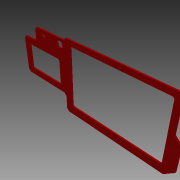
# Autodesk Inventor part: front_panel_frame
Saved by Autodesk Inventor 2014 (Build 180170000, 170)
## iProperties
Created: 2014-03-23
Part Number: front_panel_frame
Material: ABS Plastic
Document SubType Name: Modeling
Designer: buben
Density: 1.06 g/cm^3
Appearance: Smooth - Red
Author: buben
Autodesk Inventor part; units mm, degrees
ref_plane "YZ Plane" through (0, 0, 0) normal (1, 0, 0) x (0, 1, 0)
ref_plane "XZ Plane" through (0, 0, 0) normal (0, 1, 0) x (-1, 0, 0)
ref_plane "XY Plane" through (0, 0, 0) normal (0, 0, 1) x (1, 0, 0)
sketch "Sketch1" plane through (0, 0, 0) normal (0, 1, 0) x (-1, 0, 0)
  line L0 (0, -41) -> (-67, -41)
  line L1 (-67, -41) -> (-67, 0)
  line L2 (-67, 0) -> (0, 0)
  line L3 (0, 0) -> (0, -41)
  line L4 (-90, -68) -> (-242, -68)
  line L5 (-242, -68) -> (-242, 28)
  line L6 (-242, 28) -> (-90, 28)
  line L7 (-90, 28) -> (-90, -68)
  line L8 (11, -47.5) -> (11, 6.5)
  line L9 (7, 10.5) -> (-74, 10.5)
  line L10 (-78, 14.5) -> (-78, 32.5)
  line L11 (-82, 36.5) -> (-246, 36.5)
  line L12 (-250, 32.5) -> (-250, -77.5)
  line L13 (-246, -81.5) -> (-82, -81.5)
  line L14 (-78, -77.5) -> (-78, -55.5)
  line L15 (-74, -51.5) -> (7, -51.5)
  line L16 (11, -47.5) -> (7, -51.5)
  line L17 (-74, -51.5) -> (-78, -55.5)
  line L18 (-78, -77.5) -> (-82, -81.5)
  line L19 (-246, -81.5) -> (-250, -77.5)
  line L20 (-250, 32.5) -> (-246, 36.5)
  line L21 (-82, 36.5) -> (-78, 32.5)
  line L22 (-78, 14.5) -> (-74, 10.5)
  line L23 (7, 10.5) -> (11, 6.5)
  line L24 (6, -46.5) -> (-73, -46.5) construction
  line L25 (-73, -46.5) -> (-73, 5.5) construction
  line L26 (-73, 5.5) -> (6, 5.5) construction
  line L27 (6, 5.5) -> (6, -46.5) construction
  line L28 (-83, -76.5) -> (-245, -76.5) construction
  line L29 (-245, -76.5) -> (-245, 31.5) construction
  line L30 (-245, 31.5) -> (-83, 31.5) construction
  line L31 (-83, 31.5) -> (-83, -76.5) construction
  point P0 (11, 10.5)
  point P1 (-78, 10.5)
  point P2 (-78, 36.5)
  point P3 (-250, 36.5)
  point P4 (-250, -81.5)
  point P5 (-78, -81.5)
  point P6 (-78, -51.5)
  point P7 (11, -51.5)
  point P8 (-33.5, -46.5)
  point P9 (-33.5, -41)
  point P10 (6, -20.5)
  point P11 (0, -20.5)
  point P12 (-83, -22.5)
  point P13 (-90, -20)
  point P14 (-164, -76.5)
  point P15 (-166, -68)
  dimension "d0" = 67
  dimension "d1" = 41
  dimension "d2" = 152
  dimension "d3" = 96
  dimension "d4" = 4
  dimension "d5" = 4
  dimension "d6" = 4
  dimension "d7" = 4
  dimension "d8" = 4
  dimension "d9" = 4
  dimension "d10" = 4
  dimension "d11" = 4
  dimension "d12" = 4
  dimension "d13" = 4
  dimension "d14" = 4
  dimension "d15" = 4
  dimension "d16" = 4
  dimension "d17" = 4
  dimension "d18" = 4
  dimension "d19" = 4
  dimension "d20" = 79
  dimension "d21" = 52
  dimension "d22" = 162
  dimension "d23" = 108
  dimension "d24" = 10
  dimension "d25" = 26
  dimension "d26" = 5
  dimension "d27" = 5
  dimension "d28" = 5
  dimension "d29" = 5
  dimension "d30" = 5
  dimension "d31" = 5
  dimension "d32" = 5
  dimension "d48" = 8.5
  dimension "d49" = 7
  constraints: 64 end point, 16 point on line, 13 parallel, 8 midpoint, 7 perpendicular, 3 horizontal, 2 collinear, 1 coincident, 1 horizontal alignment, 1 vertical alignment
  measures "d0" distance of L1.end L2.end
  measures "d1" distance of L2.end L0.start
  measures "d2" distance of L5.end L6.end
  measures "d3" distance of L6.end L4.start
  measures "d4" distance of L8.start point (11, -51.5)
  measures "d5" distance of L15.end point (11, -51.5)
  measures "d6" distance of L15.start point (-78, -51.5)
  measures "d7" distance of L14.end point (-78, -51.5)
  measures "d8" distance of L14.start point (-78, -81.5)
  measures "d9" distance of L13.end point (-78, -81.5)
  measures "d10" distance of L13.start point (-250, -81.5)
  measures "d11" distance of L12.end point (-250, -81.5)
  measures "d12" distance of L12.start point (-250, 36.5)
  measures "d13" distance of L11.end point (-250, 36.5)
  measures "d14" distance of L11.start point (-78, 36.5)
  measures "d15" distance of L10.end point (-78, 36.5)
  measures "d16" distance of L10.start point (-78, 10.5)
  measures "d17" distance of L9.end point (-78, 10.5)
  measures "d18" distance of L9.start point (11, 10.5)
  measures "d19" distance of L8.end point (11, 10.5)
  measures "d20" distance of L25.end L26.end
  measures "d21" distance of L26.end L24.start
  measures "d22" distance of L29.end L30.end
  measures "d23" distance of L30.end L28.start
  measures "d24" distance between parallel lines of L31 L25
  measures "d25" distance between parallel lines of L30 L26
  measures "d26" distance between parallel lines of L14 L31
  measures "d27" distance between parallel lines of L8 L27
  measures "d28" distance between parallel lines of L24 L15
  measures "d29" distance between parallel lines of L26 L9
  measures "d30" distance between parallel lines of L29 L12
  measures "d31" distance between parallel lines of L13 L28
  measures "d32" distance between parallel lines of L30 L11
  measures "d48" distance between parallel lines of L28 L4
  measures "d49" distance between parallel lines of L7 L31
extrude "Extrusion1" add sketch "Sketch1" along normal blind 2
sketch "Sketch2" plane through (0, 2, 0) normal (0, 1, 0) x (1, 0, 0)
  line L0 (250, -32.5) -> (250, 77.5) projected
  line L1 (78, 55.5) -> (74, 51.5) projected
  line L2 (74, 51.5) -> (-7, 51.5) projected
  line L3 (250, 77.5) -> (260, 67.5)
  line L4 (260, 67.5) -> (260, 27.5)
  line L5 (260, 27.5) -> (250, 17.5)
  line L6 (250, 77.5) -> (250, 17.5)
  dimension "d35" = 10
  dimension "d36" = 40
  constraints: 8 end point, 3 perpendicular, 1 parallel, 1 point on line
  measures "d35" distance between parallel lines of L0 L4
  measures "d36" distance of L3.end L4.end
extrude "Extrusion2" add sketch "Sketch2" against normal blind 2
sketch "Sketch3" plane through (0, 2, 0) normal (0, 1, 0) x (1, 0, 0)
  line L0 (-7, -10.5) -> (74, -10.5) projected
  line L1 (74, -10.5) -> (78, -14.5) projected
  line L2 (78, -14.5) -> (78, -32.5) projected
  line L3 (78, 55.5) -> (74, 51.5) projected
  line L4 (74, 51.5) -> (-7, 51.5) projected
  line L5 (78, -32.5) -> (22, -32.5)
  line L6 (18, -28.5) -> (18, -14.5)
  line L7 (18, -14.5) -> (14, -10.5)
  line L8 (18, -28.5) -> (22, -32.5)
  line L9 (14, -10.5) -> (74, -10.5)
  line L10 (74, -10.5) -> (78, -14.5)
  line L11 (78, -14.5) -> (78, -32.5)
  point P0 (18, -32.5)
  dimension "d39" = 4
  dimension "d40" = 4
  dimension "d41" = 4
  dimension "d42" = 60
  constraints: 14 end point, 3 perpendicular, 3 point on line, 2 collinear, 1 parallel
  measures "d39" horizontal distance of L7.end L6.end
  measures "d40" distance of L6.start point (18, -32.5)
  measures "d41" distance of L5.end point (18, -32.5)
  measures "d42" distance between parallel lines of L2 L6
extrude "Extrusion3" add sketch "Sketch3" against normal blind 2
chamfer "Chamfer1" distance 2 angle 45 8 edges at (0, 1, -41) (67, 1, -41) (90, 1, -68) (90, 1, 28) (0, 1, 0) (67, 1, 0) (242, 1, 28) (242, 1, -68)
sketch "Sketch4" plane through (0, 2, 0) normal (0, 1, 0) x (1, 0, 0)
  line L0 (18, -14.5) -> (18, -28.5) projected
  line L1 (22, -32.5) -> (78, -32.5) projected
  circle A0 centre (69.75, -23.4) radius 5.5
  circle A1 centre (50.75, -23.4) radius 1
  circle A2 centre (35.75, -23.4) radius 3
  point P0 (0, 0)
  dimension "d50" = 11
  dimension "d51" = 2
  dimension "d52" = 6
  dimension "d53" = 19
  dimension "d54" = 15
  dimension "d55" = 9.1
  dimension "d56" = 51.75
  constraints: 3 centre point, 2 horizontal alignment
  measures "d50" diameter of A0
  measures "d51" diameter of A1
  measures "d52" diameter of A2
  measures "d53" distance of A1.centre A0.centre
  measures "d54" distance of A2.centre A1.centre
  measures "d55" distance from line of L1 A0.centre
  measures "d56" distance from line of A0.centre L0
extrude "Extrusion4" cut sketch "Sketch4" against normal through all
equation "\"d5\" = d4"
equation "\"d6\" = d4"
equation "\"d7\" = d6"
equation "\"d8\" = d4"
equation "\"d9\" = d8"
equation "\"d10\" = d4"
equation "\"d11\" = d10"
equation "\"d12\" = d4"
equation "\"d13\" = d12"
equation "\"d14\" = d4"
equation "\"d15\" = d14"
equation "\"d16\" = d4"
equation "\"d17\" = d16"
equation "\"d18\" = d4"
equation "\"d19\" = d18"
equation "\"d26\" = 0.5 * d24"
equation "\"d27\" = d26"
equation "\"d28\" = d27"
equation "\"d29\" = d28"
equation "\"d30\" = d26"
equation "\"d31\" = d30"
equation "\"d32\" = d30"
equation "\"d41\" = d40"
body "Solid1"
